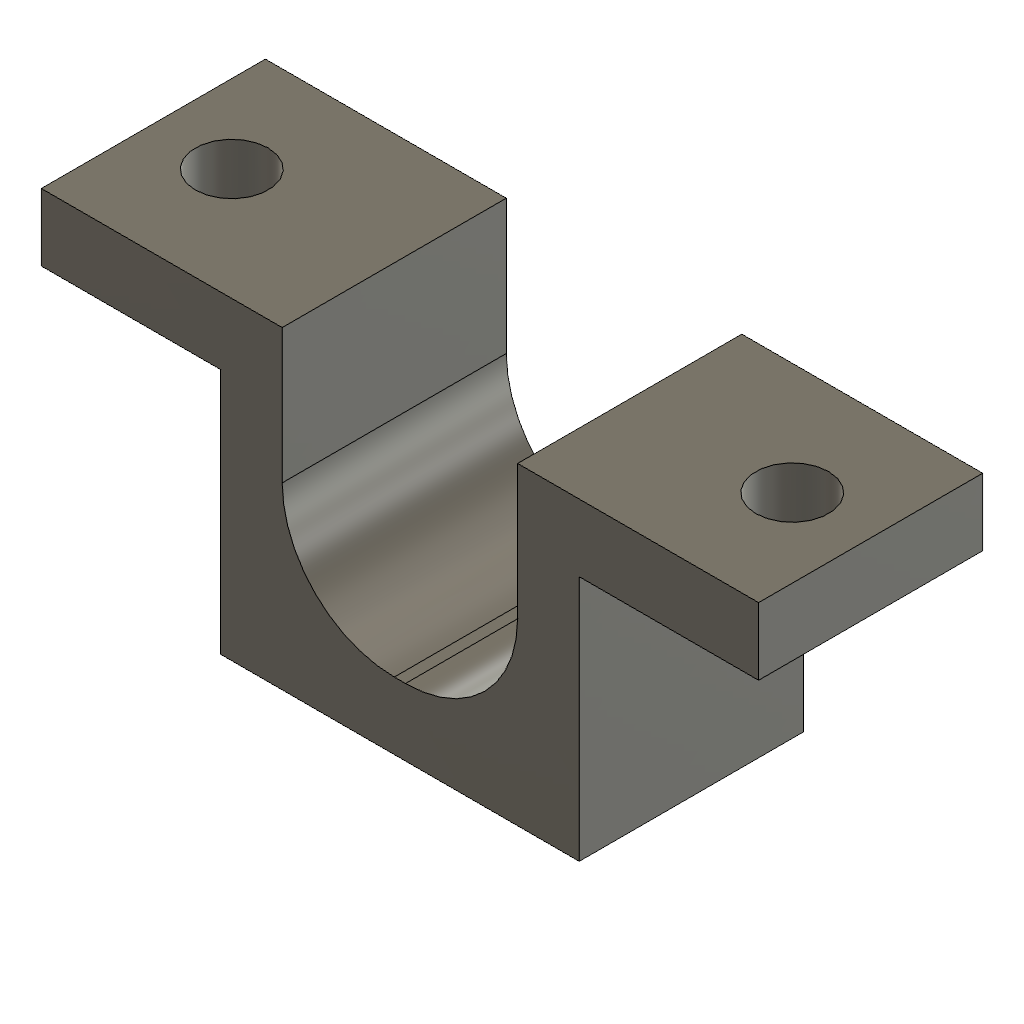
TankBot Charger Clamp (Autodesk Fusion 360 design; units mm, degrees)
Autodesk Fusion 360 part; units mm, degrees
box "BoxPrimitive1" add length 10 width 16 height 3 placed x (0, 0, 1) y (1, 0, 0) z (0, 1, 0) at (0, 0, 0)
box "BoxPrimitive2" add length 10 width 3 height 10 placed x (0, 0, -1) y (-1, 0, 0) z (0, 1, 0) at (3, 3, 10)
box "BoxPrimitive3" add length 10 width 3 height 10 placed x (0, 0, -1) y (-1, 0, 0) z (0, 1, 0) at (16, 3, 10)
box "BoxPrimitive4" add length 3 width 10 height 7 placed x (0, -1, 0) y (0, 0, -1) z (1, 0, 0) at (16, 13, 10)
box "BoxPrimitive5" add length 3 width 10 height 7 placed x (0, -1, 0) y (0, 0, 1) z (-1, 0, 0) at (0, 13, 0)
hole "Hole1" at (20.5, 10, 5) direction (0, 1, 0) diameter 3.25 depth 3 tip angle 180
hole "Hole2" at (-4.5, 10, 5) direction (0, 1, 0) diameter 3.25 depth 3 tip angle 180
extrude "Extrude1" add 1 faces at (23, 12, 3.3333) along direction (1, 0, 0) blind 1
extrude "Extrude2" add 1 faces at (-7, 12, 6.6667) along direction (-1, 0, 0) blind 1
extrude "Extrude3" add 1 faces at (14.9598, 13, 4.9595) along direction (0, 1, 0) blind 1
extrude "Extrude4" add 1 faces at (1.0402, 13, 4.9595) along direction (0, 1, 0) blind 1
extrude "Extrude5" cut 1 faces at (20.0859, 10, 1.131) along direction (0, 1, 0) blind 1
extrude "Extrude6" cut 1 faces at (-4.0859, 10, 1.131) along direction (0, 1, 0) blind 1
extrude "Extrude7" cut 1 faces at (13, 6.6667, 6.6667) along direction (1, 0, 0) blind 0.25
extrude "Extrude8" cut 1 faces at (3, 6.6667, 6.6667) along direction (-1, 0, 0) blind 0.25
fillet "Fillet3" radius 5 1 edges at (2.75, 3, 5)
fillet "Fillet4" radius 5 1 edges at (13.25, 3, 5)
